Autodesk Inventor part; units mm, degrees
(part 2 of 2)
  constraints: 312 end point, 226 point on circle, 151 symmetric about line, 118 centre point, 80 tangent, 20 parallel, 19 midpoint, 11 concentric, 5 point on line, 2 collinear, 2 vertical, 1 perpendicular, 53 other
  measures "d313" diameter of A129
extrude "Выдавливание12" cut sketch "Эскиз14" against normal blind 10 contours L66 A123 L20 L23 L26 A127 L12 | L12 A127 L30 L24 L66 | L24 L30 L86 L66 | L20 L77 L26 L23 | L20 L18 L26 L77 | L87 L78 L80 L66 | L20 A87 L45 L14 L26 L18 | A68 L27 L77 A128 L68 L29 | L68 A128 L77 L73 L50 L56 L29 | L14 L45 L17 L33 L26 | L27 A63 L32 L70 A128 L77 | L45 L36 L33 L17 | A128 L70 L32 L54 L48 L76 L73 L77 | L137 L134 L141 L126 A190 L139 | L38 L60 L63 L42 L35 | L140 L98 L94 L126 | L94 L98 A182 L95 L93 L91 A180 L126 | L93 L95 L90 L91 | L90 L95 L100 L89 L107 A158 L91 | L127 A183 L128 L99 A143 L96 A147 L97 | L89 L100 L102 L107 | L105 L123 L120 L103 L101
fillet "Сопряжение9" radius 2 9 edges at (-81.135, 1.5, -32.6639) (-59.9846, 1.5, -10.9971) (-22.6651, 1.5, -91.1362) (-14.2901, 1.5, -92.0446) (3.5996, 1.5, -74.5813) (21.0591, 1.5, -92.0446) (-82.0446, 1.5, 11.0629) (-82.0446, 1.5, -24.2901) (-64.5813, 1.5, -6.4004)
fillet "Сопряжение10" radius 2 12 edges at (10.1192, 1.5, 58.5903) (-11.5476, 1.5, 37.4399) (-33.6076, 1.5, 59.4999) (1.7454, 1.5, 59.4999) (-16.1443, 1.5, 42.0366) (47.4399, 1.5, -21.5476) (68.5915, 1.5, 0.1204) (69.4999, 1.5, -8.2546) (52.0366, 1.5, -26.1443) (69.4999, 1.5, -43.6038) (20.5079, 1.5, 59.4999) (69.4999, 1.5, 10.52)
sketch "Эскиз17" plane through (0, 3, 0) normal (0, 1, 0) x (1, 0, 0)
  line L0 (7.5288, -18.3301) -> (28.3301, 2.4712) projected
  line L1 (56.1929, -18.7322) -> (28.5794, -46.3463) projected
  line L2 (-78.6134, 20.7752) -> (-65.9616, 7.8144) projected
  arc A0 (-65.9785, 5.0031) -> (-65.9616, 7.8144) centre (-67.3927, 6.4174) ccw projected
  line L3 (-65.9785, 5.0031) -> (-78.6304, -7.6487) projected
  arc A1 (-82.0446, -6.2345) -> (-78.6304, -7.6487) centre (-80.0446, -6.2345) ccw projected
  line L4 (-82.0446, -6.2345) -> (-82.0446, 19.3781) projected
  arc A2 (-78.6134, 20.7752) -> (-82.0446, 19.3781) centre (-80.0446, 19.3781) ccw projected
  line L5 (-20.0735, 50.8748) -> (-40.8748, 30.0735) projected
  line L6 (-68.891, 51.1241) -> (-41.2769, 78.7376) projected
  line L7 (-74.128, 54.9885) -> (-84.082, 39.9808) projected
  line L8 (-29.9864, 94.0836) -> (-44.9297, 84.1856) projected
  arc A3 (-44.9297, 84.1856) -> (-45.4331, 83.7742) centre (-43.1349, 81.476) ccw projected
  line L9 (-45.4331, 83.7742) -> (-73.7176, 55.4902) projected
  arc A4 (-73.7176, 55.4902) -> (-74.128, 54.9885) centre (-71.4195, 53.192) ccw projected
  line L10 (61.6409, -22.385) -> (66.4729, -15.09) projected
  arc A5 (69.4999, -14.7276) -> (66.4729, -15.09) centre (68.1403, -16.1944) ccw projected
  arc A6 (24.7276, -59.4999) -> (69.4999, -14.7276) centre (25.7917, -15.7917) ccw projected
  arc A7 (25.082, -56.4661) -> (24.7276, -59.4999) centre (26.1874, -58.1328) ccw projected
  line L11 (25.082, -56.4661) -> (32.4438, -51.5833) projected
  arc A8 (32.4438, -51.5833) -> (32.9455, -51.1729) centre (30.6473, -48.8748) ccw projected
  line L12 (32.9455, -51.1729) -> (61.2295, -22.8884) projected
  arc A9 (61.2295, -22.8884) -> (61.6409, -22.385) centre (58.9313, -20.5902) ccw projected
  line L13 (-10.1162, -36.0085) -> (7.2688, -18.6234) projected
  line L14 (28.5794, -46.3463) -> (11.4656, -57.6973) projected
  arc A10 (8.9631, -57.4617) -> (11.4656, -57.6973) centre (10.3601, -56.0306) ccw projected
  line L15 (8.9631, -57.4617) -> (-10.0991, -38.8539) projected
  arc A11 (-10.1162, -36.0085) -> (-10.0991, -38.8539) centre (-8.702, -37.4227) ccw projected
  line L16 (28.6234, 2.7312) -> (46.0085, 20.1162) projected
  arc A12 (48.8539, 20.0991) -> (46.0085, 20.1162) centre (47.4227, 18.702) ccw projected
  line L17 (48.8539, 20.0991) -> (67.4636, 1.035) projected
  arc A13 (67.6998, -1.4665) -> (67.4636, 1.035) centre (66.0324, -0.362) ccw projected
  line L18 (67.6998, -1.4665) -> (56.5654, -18.2765) projected
  line L19 (-40.8212, 79.1101) -> (-24.0112, 90.2445) projected
  arc A14 (-21.5097, 90.0083) -> (-24.0112, 90.2445) centre (-22.9067, 88.5771) ccw projected
  line L20 (-21.5097, 90.0083) -> (-0.9971, 69.9846) projected
  line L21 (-0.9971, 69.9846) -> (-19.8135, 51.1682) projected
  line L22 (-80.242, 34.0103) -> (-68.891, 51.1241) projected
  line L23 (-41.1682, 29.8135) -> (-58.5532, 12.4285) projected
  arc A15 (-61.3986, 12.4456) -> (-58.5532, 12.4285) centre (-59.9674, 13.8427) ccw projected
  line L24 (-61.3986, 12.4456) -> (-80.0064, 31.5078) projected
  arc A16 (-80.242, 34.0103) -> (-80.0064, 31.5078) centre (-78.5753, 32.9048) ccw projected
  arc A17 (13.3479, 84.3334) -> (13.2557, 84.2373) centre (15.648, 82.0333) ccw projected
  line L25 (13.2557, 84.2373) -> (4.9969, 75.9785) projected
  arc A18 (2.1856, 75.9616) -> (4.9969, 75.9785) centre (3.5826, 77.3927) ccw projected
  line L26 (2.1856, 75.9616) -> (-10.7752, 88.6134) projected
  arc A19 (-9.3781, 92.0446) -> (-10.7752, 88.6134) centre (-9.3781, 90.0446) ccw projected
  line L27 (-9.3781, 92.0446) -> (16.2306, 92.0446) projected
  arc A20 (17.6448, 88.6304) -> (16.2306, 92.0446) centre (16.2306, 90.0446) ccw projected
  line L28 (17.6448, 88.6304) -> (13.3479, 84.3334) projected
  line L29 (53.4338, 27.5416) -> (61.6926, 35.8004) projected
  arc A21 (61.6926, 35.8004) -> (61.7887, 35.8926) centre (59.4886, 38.1927) ccw projected
  line L30 (61.7887, 35.8926) -> (66.0857, 40.1896) projected
  arc A22 (69.4999, 38.7753) -> (66.0857, 40.1896) centre (67.4999, 38.7753) ccw projected
  line L31 (69.4999, 38.7753) -> (69.4999, 13.1666) projected
  arc A23 (66.0687, 11.7696) -> (69.4999, 13.1666) centre (67.4999, 13.1666) ccw projected
  line L32 (66.0687, 11.7696) -> (53.4169, 24.7303) projected
  arc A24 (53.4338, 27.5416) -> (53.4169, 24.7303) centre (54.848, 26.1273) ccw projected
  line L33 (-30.1934, -56.0857) -> (-17.5416, -43.4338) projected
  arc A25 (-14.7303, -43.4169) -> (-17.5416, -43.4338) centre (-16.1273, -44.848) ccw projected
  line L34 (-14.7303, -43.4169) -> (-1.7696, -56.0687) projected
  arc A26 (-3.1666, -59.4999) -> (-1.7696, -56.0687) centre (-3.1666, -57.4999) ccw projected
  line L35 (-3.1666, -59.4999) -> (-28.7792, -59.4999) projected
  arc A27 (-30.1934, -56.0857) -> (-28.7792, -59.4999) centre (-28.7792, -57.4999) ccw projected
  line L36 (30.1437, 63.295) -> (40.7503, 52.6884) projected
  arc A28 (40.7503, 24.4041) -> (40.7503, 52.6884) centre (26.6081, 38.5462) ccw projected
  line L37 (40.7503, 24.4041) -> (-22.8893, -39.2355) projected
  arc A29 (-51.1736, -39.2355) -> (-22.8893, -39.2355) centre (-37.0315, -25.0934) ccw projected
  line L38 (-51.1736, -39.2355) -> (-61.7802, -28.6289) projected
  arc A30 (-61.7802, -0.3447) -> (-61.7802, -28.6289) centre (-47.6381, -14.4868) ccw projected
  line L39 (-61.7802, -0.3447) -> (1.8594, 63.295) projected
  arc A31 (30.1437, 63.295) -> (1.8594, 63.295) centre (16.0015, 49.1528) ccw projected
  circle A32 centre (47.4678, 26.1718) radius 1.5 projected
  circle A33 centre (-28.1927, -49.4886) radius 1.5 projected
  circle A34 centre (-72.0333, -5.648) radius 1.5 projected
  circle A35 centre (15.648, 82.0333) radius 1.5 projected
  circle A36 centre (59.4886, 38.1927) radius 1.5 projected
  circle A37 centre (-16.1718, -37.4678) radius 1.5 projected
  circle A38 centre (-60.0125, 6.3729) radius 1.5 projected
  circle A39 centre (3.6271, 70.0125) radius 1.5 projected
  circle A40 centre (4.9706, -16.3253) radius 1.5 projected
  circle A41 centre (-17.5154, 48.87) radius 1.5 projected
  circle A42 centre (26.3253, 5.0294) radius 1.5 projected
  circle A43 centre (-38.87, 27.5154) radius 1.5 projected
  circle A44 centre (62.3989, -52.3991) radius 1.6 projected
  circle A45 centre (-74.9438, 84.9436) radius 1.6 projected
  arc A46 (90.1213, 55.3142) -> (87.4532, 56.39) centre (88.2676, 54.5634) ccw projected
  arc A47 (33.8453, 109.9979) -> (87.4532, 56.39) centre (70.9224, 93.4671) ccw projected
  arc A48 (33.8453, 109.9979) -> (32.7695, 112.666) centre (32.0187, 110.8123) ccw projected
  arc A49 (32.7695, 112.666) -> (27.3747, 114.679) centre (-6.2724, 16.2724) ccw projected
  arc A50 (27.3747, 114.679) -> (24.7276, 112.7866) centre (26.7276, 112.7866) ccw projected
  line L40 (24.7276, 112.7866) -> (24.7276, 103.5447) projected
  arc A51 (22.7276, 101.5447) -> (24.7276, 103.5447) centre (22.7276, 103.5447) ccw projected
  line L41 (22.7276, 101.5447) -> (-35.2724, 101.5447) projected
  arc A52 (-37.2724, 103.5447) -> (-35.2724, 101.5447) centre (-35.2724, 103.5447) ccw projected
  line L42 (-37.2724, 103.5447) -> (-37.2724, 112.7866) projected
  arc A53 (-37.2724, 112.7866) -> (-39.9194, 114.679) centre (-39.2724, 112.7866) ccw projected
  arc A54 (-39.9194, 114.679) -> (-104.679, 49.9194) centre (-6.2724, 16.2724) ccw projected
  arc A55 (-104.679, 49.9194) -> (-102.7866, 47.2724) centre (-102.7866, 49.2724) ccw projected
  line L43 (-102.7866, 47.2724) -> (-93.5447, 47.2724) projected
  arc A56 (-91.5447, 45.2724) -> (-93.5447, 47.2724) centre (-93.5447, 45.2724) ccw projected
  line L44 (-91.5447, 45.2724) -> (-91.5447, -12.7276) projected
  arc A57 (-93.5447, -14.7276) -> (-91.5447, -12.7276) centre (-93.5447, -12.7276) ccw projected
  line L45 (-93.5447, -14.7276) -> (-102.7866, -14.7276) projected
  arc A58 (-102.7866, -14.7276) -> (-104.679, -17.3747) centre (-102.7866, -16.7276) ccw projected
  arc A59 (-104.679, -17.3747) -> (-101.9399, -24.5163) centre (-6.2724, 16.2724) ccw projected
  arc A60 (-101.9399, -24.5163) -> (-100.0204, -25.7303) centre (-100.1002, -23.7319) ccw projected
  arc A61 (-48.275, -77.4757) -> (-100.0204, -25.7303) centre (-98.035, -75.4903) ccw projected
  arc A62 (-48.275, -77.4757) -> (-47.061, -79.3952) centre (-46.2766, -77.5555) ccw projected
  arc A63 (-47.061, -79.3952) -> (-39.9194, -82.1343) centre (-6.2724, 16.2724) ccw projected
  arc A64 (-39.9194, -82.1343) -> (-37.2724, -80.2419) centre (-39.2724, -80.2419) ccw projected
  line L46 (-37.2724, -80.2419) -> (-37.2724, -71) projected
  arc A65 (-35.2724, -69) -> (-37.2724, -71) centre (-35.2724, -71) ccw projected
  line L47 (-35.2724, -69) -> (22.7276, -69) projected
  arc A66 (24.7276, -71) -> (22.7276, -69) centre (22.7276, -71) ccw projected
  line L48 (24.7276, -71) -> (24.7276, -80.2419) projected
  arc A67 (24.7276, -80.2419) -> (27.3747, -82.1343) centre (26.7276, -80.2419) ccw projected
  arc A68 (27.3747, -82.1343) -> (92.1343, -17.3747) centre (-6.2724, 16.2724) ccw projected
  arc A69 (92.1343, -17.3747) -> (90.2419, -14.7276) centre (90.2419, -16.7276) ccw projected
  line L49 (90.2419, -14.7276) -> (81, -14.7276) projected
  arc A70 (79, -12.7276) -> (81, -14.7276) centre (81, -12.7276) ccw projected
  line L50 (79, -12.7276) -> (79, 45.2724) projected
  arc A71 (81, 47.2724) -> (79, 45.2724) centre (81, 45.2724) ccw projected
  line L51 (81, 47.2724) -> (90.2419, 47.2724) projected
  arc A72 (90.2419, 47.2724) -> (92.1343, 49.9194) centre (90.2419, 49.2724) ccw projected
  arc A73 (92.1343, 49.9194) -> (90.1213, 55.3142) centre (-6.2724, 16.2724) ccw projected
  circle A74 centre (-94.1551, 63.85) radius 1.5 projected
  circle A75 centre (41.3053, -71.6104) radius 1.5 projected
  circle A76 centre (81.6104, -31.3053) radius 1.5 projected
  circle A77 centre (-53.85, 104.1551) radius 1.5 projected
  circle A78 centre (-83.0755, 76.8119) radius 1.5 projected
  circle A79 centre (54.2672, -60.5308) radius 1.5 projected
  circle A80 centre (70.5306, -44.2673) radius 1.5 projected
  circle A81 centre (-66.812, 93.0753) radius 1.5 projected
  circle A82 centre (-45.0925, -54.9329) radius 1.5 projected
  circle A83 centre (59.1841, 49.909) radius 1.5 projected
  circle A84 centre (-43.1349, 81.476) radius 1.5 projected
  circle A85 centre (29.7645, -47.992) radius 1.5 projected
  circle A86 centre (-77.6194, -22.406) radius 1.5 projected
  circle A87 centre (27.3717, 81.7363) radius 1.5 projected
  circle A88 centre (-71.4195, 53.192) radius 1.5 projected
  circle A89 centre (58.0485, -19.7074) radius 1.5 projected
  circle A90 centre (-85.2947, 0.2724) radius 1.5 projected
  circle A91 centre (72.75, 0.2724) radius 1.5 projected
  circle A92 centre (-22.2724, 95.2947) radius 1.5 projected
  circle A93 centre (9.7276, -62.75) radius 1.5 projected
  circle A94 centre (-85.2947, 32.2724) radius 1.5 projected
  circle A95 centre (72.75, 32.2724) radius 1.5 projected
  circle A96 centre (9.7276, 95.2947) radius 1.5 projected
  circle A97 centre (-22.2724, -62.75) radius 1.5 projected
  circle A98 centre (-72.0333, -5.648) radius 1.5 projected
  circle A99 centre (-28.1927, -49.4886) radius 1.5 projected
  line L52 (-72.0333, -5.648) -> (-28.1927, -49.4886)
  line L53 (-28.1927, -49.4886) -> (-6.3904, -27.6864)
  line L54 (-6.3904, -27.6864) -> (-50.2311, 16.1543)
  line L55 (-50.2311, 16.1543) -> (-72.0333, -5.648)
  circle A100 centre (-50.2311, 16.1543) radius 1.5
  circle A101 centre (-6.3904, -27.6864) radius 1.5
  arc A102 (7.2688, -18.6234) -> (7.5288, -18.3301) centre (4.9706, -16.3253) ccw projected
  arc A103 (28.3301, 2.4712) -> (28.6234, 2.7312) centre (26.3253, 5.0294) ccw projected
  arc A104 (56.5654, -18.2765) -> (56.1929, -18.7322) centre (58.9313, -20.5902) ccw projected
  line L56 (-84.082, 39.9808) -> (-90.5571, 63.0573) projected
  line L57 (-90.5571, 63.0573) -> (-80.7117, 74.5752) projected
  line L58 (-80.7117, 74.5752) -> (-64.6017, 90.6852) projected
  line L59 (-64.6017, 90.6852) -> (-53.0539, 100.5561) projected
  line L60 (-53.0539, 100.5561) -> (-29.9864, 94.0836) projected
  arc A105 (-41.2769, 78.7376) -> (-40.8212, 79.1101) centre (-43.1349, 81.476) ccw projected
  arc A106 (-19.8135, 51.1682) -> (-20.0735, 50.8748) centre (-17.5154, 48.87) ccw projected
  arc A107 (-40.8748, 30.0735) -> (-41.1682, 29.8135) centre (-38.87, 27.5154) ccw projected
  dimension "d339" = 30.833
  dimension "d340" = 3
  dimension "d341" = 3
  constraints: 8 end point, 2 centre point, 2 coincident, 2 parallel, 1 perpendicular
  measures "d339" distance of L53.end L52.end
  measures "d340" diameter of A100
  measures "d341" diameter of A101
extrude "Выдавливание13" cut sketch "Эскиз17" against normal blind 10 contours A100 L55 L54 | L54 L55 A100 | A101 L53 L54 | L54 L53 A101
sketch "Эскиз18" plane through (0, 3, 0) normal (0, 1, 0) x (1, 0, 0)
  circle A0 centre (-6.3904, -27.6864) radius 1.5 projected
  circle A1 centre (-50.2311, 16.1543) radius 1.5 projected
  line L0 (8.9631, -57.4617) -> (-10.0991, -38.8539) projected
  arc A2 (-10.1162, -36.0085) -> (-10.0991, -38.8539) centre (-8.702, -37.4227) ccw projected
  line L1 (-10.1162, -36.0085) -> (7.2688, -18.6234) projected
  arc A3 (7.2688, -18.6234) -> (7.5288, -18.3301) centre (4.9706, -16.3253) ccw projected
  line L2 (7.5288, -18.3301) -> (28.3301, 2.4712) projected
  arc A4 (28.3301, 2.4712) -> (28.6234, 2.7312) centre (26.3253, 5.0294) ccw projected
  line L3 (28.6234, 2.7312) -> (46.0085, 20.1162) projected
  arc A5 (48.8539, 20.0991) -> (46.0085, 20.1162) centre (47.4227, 18.702) ccw projected
  line L4 (48.8539, 20.0991) -> (67.4636, 1.035) projected
  arc A6 (67.6998, -1.4665) -> (67.4636, 1.035) centre (66.0324, -0.362) ccw projected
  line L5 (67.6998, -1.4665) -> (56.5654, -18.2765) projected
  arc A7 (56.5654, -18.2765) -> (56.1929, -18.7322) centre (58.9313, -20.5902) ccw projected
  line L6 (56.1929, -18.7322) -> (28.5794, -46.3463) projected
  line L7 (28.5794, -46.3463) -> (11.4656, -57.6973) projected
  arc A8 (8.9631, -57.4617) -> (11.4656, -57.6973) centre (10.3601, -56.0306) ccw projected
  arc A9 (-73.7176, 55.4902) -> (-74.128, 54.9885) centre (-71.4195, 53.192) ccw projected
  line L8 (-74.128, 54.9885) -> (-84.082, 39.9808) projected
  line L9 (-84.082, 39.9808) -> (-90.5571, 63.0573) projected
  line L10 (-90.5571, 63.0573) -> (-80.7117, 74.5752) projected
  line L11 (-80.7117, 74.5752) -> (-64.6017, 90.6852) projected
  line L12 (-64.6017, 90.6852) -> (-53.0539, 100.5561) projected
  line L13 (-53.0539, 100.5561) -> (-29.9864, 94.0836) projected
  line L14 (-29.9864, 94.0836) -> (-44.9297, 84.1856) projected
  arc A10 (-44.9297, 84.1856) -> (-45.4331, 83.7742) centre (-43.1349, 81.476) ccw projected
  line L15 (-45.4331, 83.7742) -> (-73.7176, 55.4902) projected
  line L16 (-78.6134, 20.7752) -> (-65.9616, 7.8144) projected
  arc A11 (-65.9785, 5.0031) -> (-65.9616, 7.8144) centre (-67.3927, 6.4174) ccw projected
  line L17 (-65.9785, 5.0031) -> (-78.6304, -7.6487) projected
  arc A12 (-82.0446, -6.2345) -> (-78.6304, -7.6487) centre (-80.0446, -6.2345) ccw projected
  line L18 (-82.0446, -6.2345) -> (-82.0446, 19.3781) projected
  arc A13 (-78.6134, 20.7752) -> (-82.0446, 19.3781) centre (-80.0446, 19.3781) ccw projected
  line L19 (61.6409, -22.385) -> (66.4729, -15.09) projected
  arc A14 (69.4999, -14.7276) -> (66.4729, -15.09) centre (68.1403, -16.1944) ccw projected
  arc A15 (24.7276, -59.4999) -> (69.4999, -14.7276) centre (25.7917, -15.7917) ccw projected
  arc A16 (25.082, -56.4661) -> (24.7276, -59.4999) centre (26.1874, -58.1328) ccw projected
  line L20 (25.082, -56.4661) -> (32.4438, -51.5833) projected
  arc A17 (32.4438, -51.5833) -> (32.9455, -51.1729) centre (30.6473, -48.8748) ccw projected
  line L21 (32.9455, -51.1729) -> (61.2295, -22.8884) projected
  arc A18 (61.2295, -22.8884) -> (61.6409, -22.385) centre (58.9313, -20.5902) ccw projected
  line L22 (53.4338, 27.5416) -> (61.6926, 35.8004) projected
  arc A19 (61.6926, 35.8004) -> (61.7887, 35.8926) centre (59.4886, 38.1927) ccw projected
  line L23 (61.7887, 35.8926) -> (66.0857, 40.1896) projected
  arc A20 (69.4999, 38.7753) -> (66.0857, 40.1896) centre (67.4999, 38.7753) ccw projected
  line L24 (69.4999, 38.7753) -> (69.4999, 13.1666) projected
  arc A21 (66.0687, 11.7696) -> (69.4999, 13.1666) centre (67.4999, 13.1666) ccw projected
  line L25 (66.0687, 11.7696) -> (53.4169, 24.7303) projected
  arc A22 (53.4338, 27.5416) -> (53.4169, 24.7303) centre (54.848, 26.1273) ccw projected
  arc A23 (13.3479, 84.3334) -> (13.2557, 84.2373) centre (15.648, 82.0333) ccw projected
  line L26 (13.2557, 84.2373) -> (4.9969, 75.9785) projected
  arc A24 (2.1856, 75.9616) -> (4.9969, 75.9785) centre (3.5826, 77.3927) ccw projected
  line L27 (2.1856, 75.9616) -> (-10.7752, 88.6134) projected
  arc A25 (-9.3781, 92.0446) -> (-10.7752, 88.6134) centre (-9.3781, 90.0446) ccw projected
  line L28 (-9.3781, 92.0446) -> (16.2306, 92.0446) projected
  arc A26 (17.6448, 88.6304) -> (16.2306, 92.0446) centre (16.2306, 90.0446) ccw projected
  line L29 (17.6448, 88.6304) -> (13.3479, 84.3334) projected
  arc A27 (-41.2769, 78.7376) -> (-40.8212, 79.1101) centre (-43.1349, 81.476) ccw projected
  line L30 (-40.8212, 79.1101) -> (-24.0112, 90.2445) projected
  arc A28 (-21.5097, 90.0083) -> (-24.0112, 90.2445) centre (-22.9067, 88.5771) ccw projected
  line L31 (-21.5097, 90.0083) -> (-0.9971, 69.9846) projected
  line L32 (-0.9971, 69.9846) -> (-19.8135, 51.1682) projected
  arc A29 (-19.8135, 51.1682) -> (-20.0735, 50.8748) centre (-17.5154, 48.87) ccw projected
  line L33 (-20.0735, 50.8748) -> (-40.8748, 30.0735) projected
  arc A30 (-40.8748, 30.0735) -> (-41.1682, 29.8135) centre (-38.87, 27.5154) ccw projected
  line L34 (-41.1682, 29.8135) -> (-58.5532, 12.4285) projected
  arc A31 (-61.3986, 12.4456) -> (-58.5532, 12.4285) centre (-59.9674, 13.8427) ccw projected
  line L35 (-61.3986, 12.4456) -> (-80.0064, 31.5078) projected
  arc A32 (-80.242, 34.0103) -> (-80.0064, 31.5078) centre (-78.5753, 32.9048) ccw projected
  line L36 (-80.242, 34.0103) -> (-68.891, 51.1241) projected
  line L37 (-68.891, 51.1241) -> (-41.2769, 78.7376) projected
  line L38 (-30.1934, -56.0857) -> (-17.5416, -43.4338) projected
  arc A33 (-14.7303, -43.4169) -> (-17.5416, -43.4338) centre (-16.1273, -44.848) ccw projected
  line L39 (-14.7303, -43.4169) -> (-1.7696, -56.0687) projected
  arc A34 (-3.1666, -59.4999) -> (-1.7696, -56.0687) centre (-3.1666, -57.4999) ccw projected
  line L40 (-3.1666, -59.4999) -> (-28.7792, -59.4999) projected
  arc A35 (-30.1934, -56.0857) -> (-28.7792, -59.4999) centre (-28.7792, -57.4999) ccw projected
  line L41 (30.1437, 63.295) -> (40.7503, 52.6884) projected
  arc A36 (40.7503, 24.4041) -> (40.7503, 52.6884) centre (26.6081, 38.5462) ccw projected
  line L42 (40.7503, 24.4041) -> (-22.8893, -39.2355) projected
  arc A37 (-51.1736, -39.2355) -> (-22.8893, -39.2355) centre (-37.0315, -25.0934) ccw projected
  line L43 (-51.1736, -39.2355) -> (-61.7802, -28.6289) projected
  arc A38 (-61.7802, -0.3447) -> (-61.7802, -28.6289) centre (-47.6381, -14.4868) ccw projected
  line L44 (-61.7802, -0.3447) -> (1.8594, 63.295) projected
  arc A39 (30.1437, 63.295) -> (1.8594, 63.295) centre (16.0015, 49.1528) ccw projected
  circle A40 centre (47.4678, 26.1718) radius 1.5 projected
  circle A41 centre (-28.1927, -49.4886) radius 1.5 projected
  circle A42 centre (-72.0333, -5.648) radius 1.5 projected
  circle A43 centre (15.648, 82.0333) radius 1.5 projected
  circle A44 centre (59.4886, 38.1927) radius 1.5 projected
  circle A45 centre (-16.1718, -37.4678) radius 1.5 projected
  circle A46 centre (-60.0125, 6.3729) radius 1.5 projected
  circle A47 centre (3.6271, 70.0125) radius 1.5 projected
  circle A48 centre (4.9706, -16.3253) radius 1.5 projected
  circle A49 centre (-17.5154, 48.87) radius 1.5 projected
  circle A50 centre (26.3253, 5.0294) radius 1.5 projected
  circle A51 centre (-38.87, 27.5154) radius 1.5 projected
  circle A52 centre (62.3989, -52.3991) radius 1.6 projected
  circle A53 centre (-74.9438, 84.9436) radius 1.6 projected
  arc A54 (90.1213, 55.3142) -> (87.4532, 56.39) centre (88.2676, 54.5634) ccw projected
  arc A55 (33.8453, 109.9979) -> (87.4532, 56.39) centre (70.9224, 93.4671) ccw projected
  arc A56 (33.8453, 109.9979) -> (32.7695, 112.666) centre (32.0187, 110.8123) ccw projected
  arc A57 (32.7695, 112.666) -> (27.3747, 114.679) centre (-6.2724, 16.2724) ccw projected
  arc A58 (27.3747, 114.679) -> (24.7276, 112.7866) centre (26.7276, 112.7866) ccw projected
  line L45 (24.7276, 112.7866) -> (24.7276, 103.5447) projected
  arc A59 (22.7276, 101.5447) -> (24.7276, 103.5447) centre (22.7276, 103.5447) ccw projected
  line L46 (22.7276, 101.5447) -> (-35.2724, 101.5447) projected
  arc A60 (-37.2724, 103.5447) -> (-35.2724, 101.5447) centre (-35.2724, 103.5447) ccw projected
  line L47 (-37.2724, 103.5447) -> (-37.2724, 112.7866) projected
  arc A61 (-37.2724, 112.7866) -> (-39.9194, 114.679) centre (-39.2724, 112.7866) ccw projected
  arc A62 (-39.9194, 114.679) -> (-104.679, 49.9194) centre (-6.2724, 16.2724) ccw projected
  arc A63 (-104.679, 49.9194) -> (-102.7866, 47.2724) centre (-102.7866, 49.2724) ccw projected
  line L48 (-102.7866, 47.2724) -> (-93.5447, 47.2724) projected
  arc A64 (-91.5447, 45.2724) -> (-93.5447, 47.2724) centre (-93.5447, 45.2724) ccw projected
  line L49 (-91.5447, 45.2724) -> (-91.5447, -12.7276) projected
  arc A65 (-93.5447, -14.7276) -> (-91.5447, -12.7276) centre (-93.5447, -12.7276) ccw projected
  line L50 (-93.5447, -14.7276) -> (-102.7866, -14.7276) projected
  arc A66 (-102.7866, -14.7276) -> (-104.679, -17.3747) centre (-102.7866, -16.7276) ccw projected
  arc A67 (-104.679, -17.3747) -> (-101.9399, -24.5163) centre (-6.2724, 16.2724) ccw projected
  arc A68 (-101.9399, -24.5163) -> (-100.0204, -25.7303) centre (-100.1002, -23.7319) ccw projected
  arc A69 (-48.275, -77.4757) -> (-100.0204, -25.7303) centre (-98.035, -75.4903) ccw projected
  arc A70 (-48.275, -77.4757) -> (-47.061, -79.3952) centre (-46.2766, -77.5555) ccw projected
  arc A71 (-47.061, -79.3952) -> (-39.9194, -82.1343) centre (-6.2724, 16.2724) ccw projected
  arc A72 (-39.9194, -82.1343) -> (-37.2724, -80.2419) centre (-39.2724, -80.2419) ccw projected
  line L51 (-37.2724, -80.2419) -> (-37.2724, -71) projected
  arc A73 (-35.2724, -69) -> (-37.2724, -71) centre (-35.2724, -71) ccw projected
  line L52 (-35.2724, -69) -> (22.7276, -69) projected
  arc A74 (24.7276, -71) -> (22.7276, -69) centre (22.7276, -71) ccw projected
  line L53 (24.7276, -71) -> (24.7276, -80.2419) projected
  arc A75 (24.7276, -80.2419) -> (27.3747, -82.1343) centre (26.7276, -80.2419) ccw projected
  arc A76 (27.3747, -82.1343) -> (92.1343, -17.3747) centre (-6.2724, 16.2724) ccw projected
  arc A77 (92.1343, -17.3747) -> (90.2419, -14.7276) centre (90.2419, -16.7276) ccw projected
  line L54 (90.2419, -14.7276) -> (81, -14.7276) projected
  arc A78 (79, -12.7276) -> (81, -14.7276) centre (81, -12.7276) ccw projected
  line L55 (79, -12.7276) -> (79, 45.2724) projected
  arc A79 (81, 47.2724) -> (79, 45.2724) centre (81, 45.2724) ccw projected
  line L56 (81, 47.2724) -> (90.2419, 47.2724) projected
  arc A80 (90.2419, 47.2724) -> (92.1343, 49.9194) centre (90.2419, 49.2724) ccw projected
  arc A81 (92.1343, 49.9194) -> (90.1213, 55.3142) centre (-6.2724, 16.2724) ccw projected
  circle A82 centre (-94.1551, 63.85) radius 1.5 projected
  circle A83 centre (41.3053, -71.6104) radius 1.5 projected
  circle A84 centre (81.6104, -31.3053) radius 1.5 projected
  circle A85 centre (-53.85, 104.1551) radius 1.5 projected
  circle A86 centre (-83.0755, 76.8119) radius 1.5 projected
  circle A87 centre (54.2672, -60.5308) radius 1.5 projected
  circle A88 centre (70.5306, -44.2673) radius 1.5 projected
  circle A89 centre (-66.812, 93.0753) radius 1.5 projected
  circle A90 centre (-45.0925, -54.9329) radius 1.5 projected
  circle A91 centre (59.1841, 49.909) radius 1.5 projected
  circle A92 centre (-43.1349, 81.476) radius 1.5 projected
  circle A93 centre (29.7645, -47.992) radius 1.5 projected
  circle A94 centre (-77.6194, -22.406) radius 1.5 projected
  circle A95 centre (27.3717, 81.7363) radius 1.5 projected
  circle A96 centre (-71.4195, 53.192) radius 1.5 projected
  circle A97 centre (58.0485, -19.7074) radius 1.5 projected
  circle A98 centre (-85.2947, 0.2724) radius 1.5 projected
  circle A99 centre (72.75, 0.2724) radius 1.5 projected
  circle A100 centre (-22.2724, 95.2947) radius 1.5 projected
  circle A101 centre (9.7276, -62.75) radius 1.5 projected
  circle A102 centre (-85.2947, 32.2724) radius 1.5 projected
  circle A103 centre (72.75, 32.2724) radius 1.5 projected
  circle A104 centre (9.7276, 95.2947) radius 1.5 projected
  circle A105 centre (-22.2724, -62.75) radius 1.5 projected
  circle A106 centre (-17.5154, 48.87) radius 1.5 projected
  line L57 (-17.5154, 48.87) -> (-12.212, 54.1733)
  line L58 (-17.5154, 48.87) -> (-10.0154, 48.87) construction
  line L59 (-10.0154, 51.4202) -> (-20.622, 40.8136)
  line L60 (-20.622, 40.8136) -> (-25.378, 45.5696)
  line L61 (-25.378, 45.5696) -> (-14.7714, 56.1762)
  line L62 (-14.7714, 56.1762) -> (-10.0154, 51.4202)
  line L63 (-6.2724, 16.2724) -> (-50.4043, 60.4043)
  line L64 (-50.4043, 60.4043) -> (41.3053, -31.3053)
  line L65 (-6.2724, 16.2724) -> (33.6315, 56.1762)
  line L66 (33.6315, 56.1762) -> (32.7695, 55.3142)
  line L67 (32.7695, 55.3142) -> (-43.7521, -21.2074)
  arc A107 (28.3301, 2.4712) -> (28.6234, 2.7312) centre (26.3253, 5.0294) ccw
  circle A108 centre (26.3253, 5.0294) radius 1.5
  circle A109 centre (26.3253, 5.0294) radius 1.5
  line L68 (26.3253, 5.0294) -> (31.6286, 10.3327)
  line L69 (26.3253, 5.0294) -> (26.3253, 12.5294) construction
  line L70 (28.8755, 12.5294) -> (18.2689, 1.9228)
  line L71 (18.2689, 1.9228) -> (23.0249, -2.8332)
  line L72 (23.0249, -2.8332) -> (33.6315, 7.7734)
  line L73 (33.6315, 7.7734) -> (28.8755, 12.5294)
  arc A110 (7.2688, -18.6234) -> (7.5288, -18.3301) centre (4.9706, -16.3253) ccw
  circle A111 centre (4.9706, -16.3253) radius 1.5
  line L74 (2.2266, -23.6315) -> (-2.5294, -18.8755)
  line L75 (4.9706, -16.3253) -> (-2.5294, -16.3253) construction
  line L76 (4.9706, -16.3253) -> (-0.3327, -21.6286)
  arc A112 (7.2688, -18.6234) -> (7.5288, -18.3301) centre (4.9706, -16.3253) ccw
  circle A113 centre (4.9706, -16.3253) radius 1.5
  circle A114 centre (4.9706, -16.3253) radius 1.5
  line L77 (12.8332, -13.0249) -> (2.2266, -23.6315)
  line L78 (-2.5294, -18.8755) -> (8.0772, -8.2689)
  line L79 (8.0772, -8.2689) -> (12.8332, -13.0249)
  circle A115 centre (-50.2311, 16.1543) radius 1.5
  arc A116 (-40.8748, 30.0735) -> (-41.1682, 29.8135) centre (-38.87, 27.5154) ccw
  circle A117 centre (-38.87, 27.5154) radius 1.5
  arc A118 (-40.8748, 30.0735) -> (-41.1682, 29.8135) centre (-38.87, 27.5154) ccw
  arc A119 (-40.8748, 30.0735) -> (-41.1682, 29.8135) centre (-38.87, 27.5154) ccw
  circle A120 centre (-38.87, 27.5154) radius 1.5
  line L80 (-46.1762, 24.7714) -> (-41.4202, 20.0154)
  line L81 (-38.87, 27.5154) -> (-38.87, 20.0154) construction
  circle A121 centre (-38.87, 27.5154) radius 1.5
  circle A122 centre (-38.87, 27.5154) radius 1.5
  line L82 (-35.5696, 35.378) -> (-46.1762, 24.7714)
  line L83 (-30.8136, 30.622) -> (-35.5696, 35.378)
  line L84 (-41.4202, 20.0154) -> (-30.8136, 30.622)
  line L85 (-38.87, 27.5154) -> (-44.1733, 22.212)
  point P0 (0, 0)
  dimension "d344" = 7.5
  dimension "d345" = 45
  dimension "d346" = 15
  dimension "d347" = 6.726
  constraints: 58 end point, 34 symmetric about line, 16 centre point, 12 point on circle, 4 point on line, 2 parallel, 2 perpendicular, 1 equal length, 1 horizontal, 16 other
  measures "d344" distance of L57.start L57.end
  measures "d345" angle of L58 L57
  measures "d346" distance of L59.start L59.end
  measures "d347" distance of L59.end L60.end
extrude "Выдавливание14" add sketch "Эскиз18" along normal blind 4 contours L77 L74 L42 L79 L2 | L71 L42 L73 L72 L2 | L44 L80 L82 L33 L83 | L60 L33 L61 L62 L44 | A48 | A49 | A50 | A51
sketch "Эскиз19" plane through (0, 0, 0) normal (0, -1, 0) x (1, 0, 0)
  circle A0 centre (-6.3904, 27.6864) radius 1.5 projected
  circle A1 centre (-50.2311, -16.1543) radius 1.5 projected
  line L0 (-10.0991, 38.8539) -> (8.9631, 57.4617) projected
  arc A2 (11.4656, 57.6973) -> (8.9631, 57.4617) centre (10.3601, 56.0306) ccw projected
  line L1 (11.4656, 57.6973) -> (28.5794, 46.3463) projected
  line L2 (28.5794, 46.3463) -> (56.1929, 18.7322) projected
  arc A3 (56.1929, 18.7322) -> (56.5654, 18.2765) centre (58.9313, 20.5902) ccw projected
  line L3 (56.5654, 18.2765) -> (67.6998, 1.4665) projected
  arc A4 (67.4636, -1.035) -> (67.6998, 1.4665) centre (66.0324, 0.362) ccw projected
  line L4 (67.4636, -1.035) -> (48.8539, -20.0991) projected
  arc A5 (46.0085, -20.1162) -> (48.8539, -20.0991) centre (47.4227, -18.702) ccw projected
  line L5 (46.0085, -20.1162) -> (28.6234, -2.7312) projected
  arc A6 (28.6234, -2.7312) -> (28.3301, -2.4712) centre (26.3253, -5.0294) ccw projected
  line L6 (28.3301, -2.4712) -> (7.5288, 18.3301) projected
  arc A7 (7.5288, 18.3301) -> (7.2688, 18.6234) centre (4.9706, 16.3253) ccw projected
  line L7 (7.2688, 18.6234) -> (-10.1162, 36.0085) projected
  arc A8 (-10.0991, 38.8539) -> (-10.1162, 36.0085) centre (-8.702, 37.4227) ccw projected
  arc A9 (-74.128, -54.9885) -> (-73.7176, -55.4902) centre (-71.4195, -53.192) ccw projected
  line L8 (-73.7176, -55.4902) -> (-45.4331, -83.7742) projected
  arc A10 (-45.4331, -83.7742) -> (-44.9297, -84.1856) centre (-43.1349, -81.476) ccw projected
  line L9 (-44.9297, -84.1856) -> (-29.9864, -94.0836) projected
  line L10 (-29.9864, -94.0836) -> (-53.0539, -100.5561) projected
  line L11 (-53.0539, -100.5561) -> (-64.6017, -90.6852) projected
  line L12 (-64.6017, -90.6852) -> (-80.7117, -74.5752) projected
  line L13 (-80.7117, -74.5752) -> (-90.5571, -63.0573) projected
  line L14 (-90.5571, -63.0573) -> (-84.082, -39.9808) projected
  line L15 (-84.082, -39.9808) -> (-74.128, -54.9885) projected
  line L16 (-65.9616, -7.8144) -> (-78.6134, -20.7752) projected
  arc A11 (-82.0446, -19.3781) -> (-78.6134, -20.7752) centre (-80.0446, -19.3781) ccw projected
  line L17 (-82.0446, -19.3781) -> (-82.0446, 6.2345) projected
  arc A12 (-78.6304, 7.6487) -> (-82.0446, 6.2345) centre (-80.0446, 6.2345) ccw projected
  line L18 (-78.6304, 7.6487) -> (-65.9785, -5.0031) projected
  arc A13 (-65.9616, -7.8144) -> (-65.9785, -5.0031) centre (-67.3927, -6.4174) ccw projected
  line L19 (66.4729, 15.09) -> (61.6409, 22.385) projected
  arc A14 (61.6409, 22.385) -> (61.2295, 22.8884) centre (58.9313, 20.5902) ccw projected
  line L20 (61.2295, 22.8884) -> (32.9455, 51.1729) projected
  arc A15 (32.9455, 51.1729) -> (32.4438, 51.5833) centre (30.6473, 48.8748) ccw projected
  line L21 (32.4438, 51.5833) -> (25.082, 56.4661) projected
  arc A16 (24.7276, 59.4999) -> (25.082, 56.4661) centre (26.1874, 58.1328) ccw projected
  arc A17 (69.4999, 14.7276) -> (24.7276, 59.4999) centre (25.7917, 15.7917) ccw projected
  arc A18 (66.4729, 15.09) -> (69.4999, 14.7276) centre (68.1403, 16.1944) ccw projected
  line L22 (61.6926, -35.8004) -> (53.4338, -27.5416) projected
  arc A19 (53.4169, -24.7303) -> (53.4338, -27.5416) centre (54.848, -26.1273) ccw projected
  line L23 (53.4169, -24.7303) -> (66.0687, -11.7696) projected
  arc A20 (69.4999, -13.1666) -> (66.0687, -11.7696) centre (67.4999, -13.1666) ccw projected
  line L24 (69.4999, -13.1666) -> (69.4999, -38.7753) projected
  arc A21 (66.0857, -40.1896) -> (69.4999, -38.7753) centre (67.4999, -38.7753) ccw projected
  line L25 (66.0857, -40.1896) -> (61.7887, -35.8926) projected
  arc A22 (61.7887, -35.8926) -> (61.6926, -35.8004) centre (59.4886, -38.1927) ccw projected
  arc A23 (13.2557, -84.2373) -> (13.3479, -84.3334) centre (15.648, -82.0333) ccw projected
  line L26 (13.3479, -84.3334) -> (17.6448, -88.6304) projected
  arc A24 (16.2306, -92.0446) -> (17.6448, -88.6304) centre (16.2306, -90.0446) ccw projected
  line L27 (16.2306, -92.0446) -> (-9.3781, -92.0446) projected
  arc A25 (-10.7752, -88.6134) -> (-9.3781, -92.0446) centre (-9.3781, -90.0446) ccw projected
  line L28 (-10.7752, -88.6134) -> (2.1856, -75.9616) projected
  arc A26 (4.9969, -75.9785) -> (2.1856, -75.9616) centre (3.5826, -77.3927) ccw projected
  line L29 (4.9969, -75.9785) -> (13.2557, -84.2373) projected
  arc A27 (-40.8212, -79.1101) -> (-41.2769, -78.7376) centre (-43.1349, -81.476) ccw projected
  line L30 (-41.2769, -78.7376) -> (-68.891, -51.1241) projected
  line L31 (-68.891, -51.1241) -> (-80.242, -34.0103) projected
  arc A28 (-80.0064, -31.5078) -> (-80.242, -34.0103) centre (-78.5753, -32.9048) ccw projected
  line L32 (-80.0064, -31.5078) -> (-61.3986, -12.4456) projected
  arc A29 (-58.5532, -12.4285) -> (-61.3986, -12.4456) centre (-59.9674, -13.8427) ccw projected
  line L33 (-58.5532, -12.4285) -> (-41.1682, -29.8135) projected
  arc A30 (-41.1682, -29.8135) -> (-40.8748, -30.0735) centre (-38.87, -27.5154) ccw projected
  line L34 (-40.8748, -30.0735) -> (-20.0735, -50.8748) projected
  arc A31 (-20.0735, -50.8748) -> (-19.8135, -51.1682) centre (-17.5154, -48.87) ccw projected
  line L35 (-19.8135, -51.1682) -> (-0.9971, -69.9846) projected
  line L36 (-0.9971, -69.9846) -> (-21.5097, -90.0083) projected
  arc A32 (-24.0112, -90.2445) -> (-21.5097, -90.0083) centre (-22.9067, -88.5771) ccw projected
  line L37 (-24.0112, -90.2445) -> (-40.8212, -79.1101) projected
  line L38 (-17.5416, 43.4338) -> (-30.1934, 56.0857) projected
  arc A33 (-28.7792, 59.4999) -> (-30.1934, 56.0857) centre (-28.7792, 57.4999) ccw projected
  line L39 (-28.7792, 59.4999) -> (-3.1666, 59.4999) projected
  arc A34 (-1.7696, 56.0687) -> (-3.1666, 59.4999) centre (-3.1666, 57.4999) ccw projected
  line L40 (-1.7696, 56.0687) -> (-14.7303, 43.4169) projected
  arc A35 (-17.5416, 43.4338) -> (-14.7303, 43.4169) centre (-16.1273, 44.848) ccw projected
  line L41 (40.7503, -52.6884) -> (30.1437, -63.295) projected
  arc A36 (1.8594, -63.295) -> (30.1437, -63.295) centre (16.0015, -49.1528) ccw projected
  line L42 (1.8594, -63.295) -> (-61.7802, 0.3447) projected
  arc A37 (-61.7802, 28.6289) -> (-61.7802, 0.3447) centre (-47.6381, 14.4868) ccw projected
  line L43 (-61.7802, 28.6289) -> (-51.1736, 39.2355) projected
  arc A38 (-22.8893, 39.2355) -> (-51.1736, 39.2355) centre (-37.0315, 25.0934) ccw projected
  line L44 (-22.8893, 39.2355) -> (40.7503, -24.4041) projected
  arc A39 (40.7503, -52.6884) -> (40.7503, -24.4041) centre (26.6081, -38.5462) ccw projected
  circle A40 centre (47.4678, -26.1718) radius 1.5 projected
  circle A41 centre (-28.1927, 49.4886) radius 1.5 projected
  circle A42 centre (-72.0333, 5.648) radius 1.5 projected
  circle A43 centre (15.648, -82.0333) radius 1.5 projected
  circle A44 centre (59.4886, -38.1927) radius 1.5 projected
  circle A45 centre (-16.1718, 37.4678) radius 1.5 projected
  circle A46 centre (-60.0125, -6.3729) radius 1.5 projected
  circle A47 centre (3.6271, -70.0125) radius 1.5 projected
  circle A48 centre (4.9706, 16.3253) radius 1.5 projected
  circle A49 centre (-17.5154, -48.87) radius 1.5 projected
  circle A50 centre (26.3253, -5.0294) radius 1.5 projected
  circle A51 centre (-38.87, -27.5154) radius 1.5 projected
  circle A52 centre (62.3989, 52.3991) radius 1.6 projected
  circle A53 centre (-74.9438, -84.9436) radius 1.6 projected
  arc A54 (87.4532, -56.39) -> (90.1213, -55.3142) centre (88.2676, -54.5634) ccw projected
  arc A55 (90.1213, -55.3142) -> (92.1343, -49.9194) centre (-6.2724, -16.2724) ccw projected
  arc A56 (92.1343, -49.9194) -> (90.2419, -47.2724) centre (90.2419, -49.2724) ccw projected
  line L45 (81, -47.2724) -> (90.2419, -47.2724) projected
  arc A57 (79, -45.2724) -> (81, -47.2724) centre (81, -45.2724) ccw projected
  line L46 (79, 12.7276) -> (79, -45.2724) projected
  arc A58 (81, 14.7276) -> (79, 12.7276) centre (81, 12.7276) ccw projected
  line L47 (90.2419, 14.7276) -> (81, 14.7276) projected
  arc A59 (90.2419, 14.7276) -> (92.1343, 17.3747) centre (90.2419, 16.7276) ccw projected
  arc A60 (92.1343, 17.3747) -> (27.3747, 82.1343) centre (-6.2724, -16.2724) ccw projected
  arc A61 (27.3747, 82.1343) -> (24.7276, 80.2419) centre (26.7276, 80.2419) ccw projected
  line L48 (24.7276, 71) -> (24.7276, 80.2419) projected
  arc A62 (22.7276, 69) -> (24.7276, 71) centre (22.7276, 71) ccw projected
  line L49 (-35.2724, 69) -> (22.7276, 69) projected
  arc A63 (-37.2724, 71) -> (-35.2724, 69) centre (-35.2724, 71) ccw projected
  line L50 (-37.2724, 80.2419) -> (-37.2724, 71) projected
  arc A64 (-37.2724, 80.2419) -> (-39.9194, 82.1343) centre (-39.2724, 80.2419) ccw projected
  arc A65 (-39.9194, 82.1343) -> (-47.061, 79.3952) centre (-6.2724, -16.2724) ccw projected
  arc A66 (-47.061, 79.3952) -> (-48.275, 77.4757) centre (-46.2766, 77.5555) ccw projected
  arc A67 (-100.0204, 25.7303) -> (-48.275, 77.4757) centre (-98.035, 75.4903) ccw projected
  arc A68 (-100.0204, 25.7303) -> (-101.9399, 24.5163) centre (-100.1002, 23.7319) ccw projected
  arc A69 (-101.9399, 24.5163) -> (-104.679, 17.3747) centre (-6.2724, -16.2724) ccw projected
  arc A70 (-104.679, 17.3747) -> (-102.7866, 14.7276) centre (-102.7866, 16.7276) ccw projected
  line L51 (-93.5447, 14.7276) -> (-102.7866, 14.7276) projected
  arc A71 (-91.5447, 12.7276) -> (-93.5447, 14.7276) centre (-93.5447, 12.7276) ccw projected
  line L52 (-91.5447, -45.2724) -> (-91.5447, 12.7276) projected
  arc A72 (-93.5447, -47.2724) -> (-91.5447, -45.2724) centre (-93.5447, -45.2724) ccw projected
  line L53 (-102.7866, -47.2724) -> (-93.5447, -47.2724) projected
  arc A73 (-102.7866, -47.2724) -> (-104.679, -49.9194) centre (-102.7866, -49.2724) ccw projected
  arc A74 (-104.679, -49.9194) -> (-39.9194, -114.679) centre (-6.2724, -16.2724) ccw projected
  arc A75 (-39.9194, -114.679) -> (-37.2724, -112.7866) centre (-39.2724, -112.7866) ccw projected
  line L54 (-37.2724, -103.5447) -> (-37.2724, -112.7866) projected
  arc A76 (-35.2724, -101.5447) -> (-37.2724, -103.5447) centre (-35.2724, -103.5447) ccw projected
  line L55 (22.7276, -101.5447) -> (-35.2724, -101.5447) projected
  arc A77 (24.7276, -103.5447) -> (22.7276, -101.5447) centre (22.7276, -103.5447) ccw projected
  line L56 (24.7276, -112.7866) -> (24.7276, -103.5447) projected
  arc A78 (24.7276, -112.7866) -> (27.3747, -114.679) centre (26.7276, -112.7866) ccw projected
  arc A79 (27.3747, -114.679) -> (32.7695, -112.666) centre (-6.2724, -16.2724) ccw projected
  arc A80 (32.7695, -112.666) -> (33.8453, -109.9979) centre (32.0187, -110.8123) ccw projected
  arc A81 (87.4532, -56.39) -> (33.8453, -109.9979) centre (70.9224, -93.4671) ccw projected
  circle A82 centre (-94.1551, -63.85) radius 1.5 projected
  circle A83 centre (41.3053, 71.6104) radius 1.5 projected
  circle A84 centre (81.6104, 31.3053) radius 1.5 projected
  circle A85 centre (-53.85, -104.1551) radius 1.5 projected
  circle A86 centre (-83.0755, -76.8119) radius 1.5 projected
  circle A87 centre (54.2672, 60.5308) radius 1.5 projected
  circle A88 centre (70.5306, 44.2673) radius 1.5 projected
  circle A89 centre (-66.812, -93.0753) radius 1.5 projected
  circle A90 centre (-45.0925, 54.9329) radius 1.5 projected
  circle A91 centre (59.1841, -49.909) radius 1.5 projected
  circle A92 centre (-43.1349, -81.476) radius 1.5 projected
  circle A93 centre (29.7645, 47.992) radius 1.5 projected
  circle A94 centre (-77.6194, 22.406) radius 1.5 projected
  circle A95 centre (27.3717, -81.7363) radius 1.5 projected
  circle A96 centre (-71.4195, -53.192) radius 1.5 projected
  circle A97 centre (58.0485, 19.7074) radius 1.5 projected
  circle A98 centre (-85.2947, -0.2724) radius 1.5 projected
  circle A99 centre (72.75, -0.2724) radius 1.5 projected
  circle A100 centre (-22.2724, -95.2947) radius 1.5 projected
  circle A101 centre (9.7276, 62.75) radius 1.5 projected
  circle A102 centre (-85.2947, -32.2724) radius 1.5 projected
  circle A103 centre (72.75, -32.2724) radius 1.5 projected
  circle A104 centre (9.7276, -95.2947) radius 1.5 projected
  circle A105 centre (-22.2724, 62.75) radius 1.5 projected
  point P0 (0, 0)
extrude "Выдавливание15" cut sketch "Эскиз19" against normal blind 12.25 contours A48 | A49 | A50 | A51
